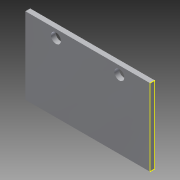
# Autodesk Inventor part: face mount
Saved by Autodesk Inventor 2013 (Build 170138000, 138)
## iProperties
Created: 2013-01-24
Part Number: face mount
Material: Aluminum 6061
Document SubType Name: Sheet Metal
Designer: Arpan
Density: 2.71 g/cm^3
Sheet Metal Rule: Default
Mass: 43.6239 g
Surface Area: 116.219 cm^2
Volume: 16.0974 cm^3
Author: Arpan
Autodesk Inventor part; units mm, degrees
ref_plane "YZ Plane" through (0, 0, 0) normal (1, 0, 0) x (0, 1, 0)
ref_plane "XZ Plane" through (0, 0, 0) normal (0, 1, 0) x (-1, 0, 0)
ref_plane "XY Plane" through (0, 0, 0) normal (0, 0, 1) x (1, 0, 0)
sketch "Sketch1" plane through (0, 0, 0) normal (0, 0, 1) x (1, 0, 0)
  line L0 (0, 0) -> (-56.9976, 0)
  line L1 (-56.9976, 50.8) -> (0, 50.8)
  line L2 (0, 50.8) -> (-7.493, 50.8)
  line L3 (-7.493, 50.8) -> (-7.493, 44.45)
  line L4 (-56.9976, 50.8) -> (-49.5046, 50.8)
  line L5 (-49.5046, 50.8) -> (-49.5046, 44.45)
  line L6 (-56.9976, 50.8) -> (-69.6976, 50.8)
  line L7 (-69.6976, 50.8) -> (-69.6976, 0)
  line L8 (-69.6976, 0) -> (-56.9976, 0)
  line L9 (0, 50.8) -> (8.89, 50.8)
  line L10 (8.89, 0) -> (0, 0)
  line L11 (0, 50.8) -> (12.7, 50.8)
  line L12 (12.7, 50.8) -> (12.7, 0)
  line L13 (12.7, 0) -> (0, 0)
  dimension "d1" = 56.9976
  dimension "d2" = 50.8
  dimension "d3" = 7.493
  dimension "d4" = 6.35
  dimension "d5" = 7.493
  dimension "d19" = 6.35
  dimension "d48" = 12.7
  dimension "d51" = 50.8
  dimension "d57" = 12.7
  constraints: 28 end point, 4 perpendicular, 3 parallel, 3 point on line, 2 collinear, 1 horizontal
  measures "d1" distance of L0.start L0.end
  measures "d2" distance of L0.end L1.start
  measures "d3" distance of L1.end L2.end
  measures "d4" distance of L2.end L3.end
  measures "d5" distance of L1.start L4.end
  measures "d19" distance of L4.end L5.end
  measures "d48" distance of L1.start L6.end
  measures "d51" distance between parallel lines of L9 L0
  measures "d57" distance of L1.end L11.end
extrude "Plate5" add sketch "Sketch1" along normal blind 3.175
sketch "Sketch6" plane through (0, 0, 3.175) normal (0, 0, 1) x (1, 0, 0)
  circle A0 centre (-7.488, 45.44) radius 3.3 projected
  circle A1 centre (-49.488, 45.44) radius 3.3 projected
  point P0 (0, 0)
extrude "Cut1" cut sketch "Sketch6" against normal blind 3.175
sketch "Sketch7" plane through (12.7, 0, 0) normal (1, 0, 0) x (0, 0, -1)
  line L0 (-3.175, 50.8) -> (-3.175, 0) projected
  line L1 (0, 0) -> (-3.175, 0) projected
  line L2 (0, 0) -> (0, 50.8) projected
  line L3 (0, 50.8) -> (-3.175, 50.8) projected
sketch "Sketch8" plane through (0, 0, 0) normal (0, 0, -1) x (-1, 0, 0)
  circle A0 centre (-5.5012, 7.9858) radius 3.2
  circle A1 centre (62.4988, 7.9858) radius 3.2
  point P0 (0, 0)
  constraints: 2 centre point, 4 other
extrude "Cut2" cut sketch "Sketch8" against normal blind 3.175
sketch "Sketch9" plane through (-69.6976, 0, 0) normal (-1, 0, 0) x (0, 0, 1)
  line L0 (3.175, 0) -> (3.175, 50.8) projected
  line L1 (0, 50.8) -> (3.175, 50.8) projected
  line L2 (0, 50.8) -> (0, 0) projected
  line L3 (0, 0) -> (3.175, 0) projected
extrude "Extrusion2" add sketch "Sketch9" along normal blind 38.1
sketch "Sketch10" plane through (0, 0, 0) normal (0, 0, -1) x (-1, 0, 0)
  line L0 (-12.7, 0) -> (107.7976, 0) projected
  line L1 (107.7976, 50.8) -> (107.7976, 0) projected
  line L2 (107.7976, 50.8) -> (107.7976, 22.225)
  line L3 (107.7976, 22.225) -> (69.6976, 22.225)
  line L4 (69.6976, 22.225) -> (69.6976, 0)
  circle A0 centre (89.254, 44.45) radius 3.3782 projected
  circle A1 centre (89.254, 28.575) radius 3.3782 projected
  point P0 (0, 0)
  dimension "d66" = 28.575
  dimension "d67" = 38.1
  constraints: 6 end point, 2 perpendicular, 2 point on line
  measures "d66" distance of L1.start L2.end
  measures "d67" distance of L2.end L3.end
extrude "Cut3" cut sketch "Sketch10" against normal blind 3.175
equation "\"d60\" = Thickness"
equation "\"d62\" = Thickness"
equation "\"d68\" = Thickness"
equation "\"BendRadius\" = Thickness"
equation "\"BendReliefWidth\" = Thickness"
equation "\"BendReliefDepth\" = 0.5 * Thickness"
equation "\"CornerReliefSize\" = 4 * Thickness"
equation "\"MinimumRemnant\" = 2 * Thickness"
equation "\"TransitionRadius\" = BendRadius"
equation "\"JacobiRadiusSize\" = BendRadius"
equation "\"GapSize\" = Thickness"
equation "\"d8\" = BendRadius"
equation "\"d56\" = BendRadius"
equation "\"Thickness\" = 3.175"
body "Solid2"
